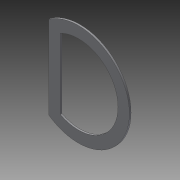
# Autodesk Inventor part: suport plate
Saved by Autodesk Inventor 2015 (Build 190159000, 159)
## iProperties
Created: 2014-07-26
Part Number: suport plate
Material: Generic
Document SubType Name: Modeling
Designer: karl
Density: 1 g/cm^3
Appearance: Default
Author: karl
Autodesk Inventor part; units mm, degrees
ref_plane "YZ Plane" through (0, 0, 0) normal (1, 0, 0) x (0, 1, 0)
ref_plane "XZ Plane" through (0, 0, 0) normal (0, 1, 0) x (-1, 0, 0)
ref_plane "XY Plane" through (0, 0, 0) normal (0, 0, 1) x (1, 0, 0)
sketch "Sketch1" plane through (0, 0, 0) normal (0, 1, 0) x (-1, 0, 0)
  circle A0 centre (0, 0) radius 90
  line L0 (55, -71.239) -> (55, 71.239)
  dimension "d0" = 180
  dimension "d1" = 55
  constraints: 2 end point, 2 point on circle, 1 centre point, 1 coincident, 1 vertical
  measures "d0" diameter of A0
  measures "d1" distance from line of L0 point (0, 0)
extrude "Extrusion1" add sketch "Sketch1" along normal blind 3 contours L0 A0 picked at (6.6667, 0)
sketch "Sketch2" plane through (0, 3, 0) normal (0, 1, 0) x (1, 0, 0)
  arc A0 (-55, -71.239) -> (-55, 71.239) centre (0, 0) ccw projected
  line L0 (-52, 73.4575) -> (-52, -73.4575)
  line L1 (-55, 71.239) -> (-55, -71.239) projected
  dimension "d4" = 3
  constraints: 2 end point, 2 point on circle, 1 vertical
  measures "d4" distance between parallel lines of L1 L0
extrude "Extrusion2" cut sketch "Sketch2" against normal blind 3 contours L1 A0 L0
sketch "Sketch3" plane through (0, 3, 0) normal (0, 1, 0) x (1, 0, 0)
  line L0 (-52, 73.4575) -> (-52, -73.4575) projected
  arc A0 (-52, -73.4575) -> (-52, 73.4575) centre (0, 0) ccw projected
  line L1 (-32, -62.2575) -> (-32, 62.2575)
  arc A1 (-32, -62.2575) -> (-32, 62.2575) centre (0, 0) ccw
  dimension "d7" = 20
  constraints: 2 end point, 2 point on circle, 1 centre point, 1 other
  measures "d7" distance between parallel lines of L0 L1
extrude "Extrusion3" cut sketch "Sketch3" against normal blind 3 contours L1 A1
sketch "Sketch4" plane through (0, 3, 0) normal (0, 1, 0) x (1, 0, 0)
  arc A0 (-32, -62.2575) -> (-32, 62.2575) centre (0, 0) ccw projected
  line L0 (51, -47.9479) -> (76.1643, -47.9479)
  line L1 (76.1643, -47.9479) -> (76.1643, 47.9479)
  line L2 (76.1643, 47.9479) -> (51, 47.9479)
  line L3 (51, 47.9479) -> (51, -47.9479)
  line L4 (-52, 73.4575) -> (-52, -73.4575) projected
  arc A1 (-52, -73.4575) -> (-52, 73.4575) centre (0, 0) ccw projected
  dimension "d10" = 103
  constraints: 8 end point, 3 point on circle, 2 parallel, 1 horizontal, 1 perpendicular
  measures "d10" distance between parallel lines of L4 L3
extrude "Extrusion4" add sketch "Sketch4" against normal blind 3 contours L3 A0
sketch "Sketch5" plane through (0, 3, 0) normal (0, 1, 0) x (1, 0, 0)
  line L0 (48, -19) -> (64, -19)
  line L1 (64, -19) -> (64, 19)
  line L2 (64, 19) -> (48, 19)
  line L3 (48, 19) -> (48, -19)
  line L4 (-52, 73.4575) -> (-52, -73.4575) projected
  point P0 (0, 0)
  point P1 (64, 0)
  dimension "d13" = 16
  dimension "d14" = 38
  dimension "d15" = 100
  constraints: 8 end point, 2 parallel, 1 horizontal, 1 horizontal alignment, 1 midpoint, 1 perpendicular
  measures "d13" distance of L2.end L1.end
  measures "d14" distance of L1.end L0.end
  measures "d15" distance between parallel lines of L4 L3
extrude "Extrusion5" cut sketch "Sketch5" against normal blind 3
sketch "Sketch6" plane through (0, 3, 0) normal (0, 1, 0) x (1, 0, 0)
  line L0 (64, -24) -> (43, -24)
  line L1 (43, -24) -> (43, 24)
  line L2 (43, 24) -> (64, 24)
  line L3 (64, 24) -> (64, -24)
  line L4 (-52, 73.4575) -> (-52, -73.4575) projected
  arc A0 (-52, -73.4575) -> (-52, 73.4575) centre (0, 0) ccw projected
  line L5 (51, 19) -> (64, 19) projected
  line L6 (64, 19) -> (64, -19) projected
  line L7 (64, -19) -> (51, -19) projected
  line L8 (51, -19) -> (51, -47.9479) projected
  arc A1 (-32, -62.2575) -> (51, -47.9479) centre (0, 0) ccw projected
  line L9 (-32, -62.2575) -> (-32, 62.2575) projected
  arc A2 (51, 47.9479) -> (-32, 62.2575) centre (0, 0) ccw projected
  line L10 (51, 47.9479) -> (51, 19) projected
  line L11 (64, -19) -> (48, -19)
  line L12 (48, -19) -> (48, 19)
  line L13 (48, 19) -> (64, 19)
  line L14 (64, 19) -> (64, -19)
  line L15 (51, 19) -> (64, 19) projected
  line L16 (64, 19) -> (64, -19) projected
  dimension "d18" = 5
  dimension "d19" = 5
  dimension "d20" = 8
  dimension "d21" = 16
  constraints: 16 end point, 4 parallel, 2 collinear, 2 horizontal, 2 perpendicular
  measures "d18" distance between parallel lines of L0 L7
  measures "d19" distance between parallel lines of L5 L2
  measures "d20" distance between parallel lines of L8 L1
  measures "d21" distance of L12.end L13.end
extrude "Extrusion6" add sketch "Sketch6" against normal blind 3 contours L0 L8 L7 L3 | L0 L1 L2 L10 L13 L12 L11 L8 | L5 L10 L2 L3
sketch "Sketch7" plane through (0, 3, 0) normal (0, 1, 0) x (1, 0, 0)
  line L0 (43, 24) -> (51, 24) projected
  line L1 (48, 24) -> (51, 24)
  line L2 (51, 24) -> (51, 60)
  line L3 (51, 60) -> (48, 60)
  line L4 (48, 60) -> (48, 24)
  line L5 (51, 47.9479) -> (51, 24) projected
  line L6 (48, 60) -> (36.0555, 60)
  line L7 (36.0555, 60) -> (36.0555, 50.951)
  line L8 (36.0555, 50.951) -> (48, 50.951)
  line L9 (48, 50.951) -> (48, 60)
  arc A0 (51, 47.9479) -> (-32, 62.2575) centre (0, 0) ccw projected
  dimension "d24" = 3
  dimension "d25" = 36
  constraints: 16 end point, 4 parallel, 2 horizontal, 2 perpendicular, 2 point on circle, 1 collinear, 1 point on line
  measures "d24" distance of L3.end L2.end
  measures "d25" distance of L2.end L1.end
extrude "Extrusion7" cut sketch "Sketch7" against normal blind 3
sketch "Sketch8" plane through (0, 3, 0) normal (0, 1, 0) x (1, 0, 0)
  line L0 (51, 60) -> (51, 24) projected
  line L1 (51, 47) -> (48, 47)
  line L2 (48, 47) -> (48, 37)
  line L3 (48, 37) -> (51, 37)
  line L4 (51, 37) -> (51, 47)
  line L5 (36.0555, 60) -> (51, 60) projected
  point P0 (0, 0)
  dimension "d28" = 3
  dimension "d29" = 10
  dimension "d30" = 13
  constraints: 8 end point, 2 parallel, 1 horizontal, 1 perpendicular, 1 point on line
  measures "d28" distance of L3.end L2.end
  measures "d29" distance of L2.end L1.end
  measures "d30" distance between parallel lines of L5 L1
extrude "Extrusion8" add sketch "Sketch8" against normal blind 3
mirror "Mirror1" about plane through (0, 0, 0) normal (0, 0, 1) of "Extrusion8", "Extrusion7"
equation "\"d19\" = d18"
body "Solid1"
